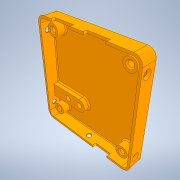
# Autodesk Inventor part: Дно корпуса электроники
Saved by Autodesk Inventor 2021.1 (Build 251245010, 245A)
## iProperties
Created: 2026-06-02
Part Number: Дно корпуса электроники
Material: Типовые
Document SubType Name: Modeling
Designer: Андрей Тарасов
Density: 1 g/cm^3
Appearance: По умолчанию
Author: Андрей Тарасов
Autodesk Inventor part; units mm, degrees
ref_plane "YZ Plane" through (0, 0, 0) normal (1, 0, 0) x (0, 1, 0)
ref_plane "XZ Plane" through (0, 0, 0) normal (0, 1, 0) x (-1, 0, 0)
ref_plane "XY Plane" through (0, 0, 0) normal (0, 0, 1) x (1, 0, 0)
sketch "Эскиз1" plane through (0, 0, 0) normal (0, 0, 1) x (1, 0, 0)
  line L0 (5, 0) -> (63.2, 0)
  line L1 (68.2, 5) -> (68.2, 65.2)
  line L2 (63.2, 70.2) -> (5, 70.2)
  line L3 (0, 65.2) -> (0, 5)
  arc A0 (5, 70.2) -> (0, 65.2) centre (5, 65.2) ccw
  arc A1 (68.2, 65.2) -> (63.2, 70.2) centre (63.2, 65.2) ccw
  arc A2 (0, 5) -> (5, 0) centre (5, 5) ccw
  arc A3 (63.2, 0) -> (68.2, 5) centre (63.2, 5) ccw
  line L4 (0, 64.1) -> (68.2, 64.1) construction
  line L5 (0, 6.1) -> (68.2, 6.1) construction
  line L6 (6.1, 70.2) -> (6.1, 0) construction
  line L7 (62.1, 70.2) -> (62.1, 0) construction
  circle A4 centre (25, 19.2) radius 1.9
  circle A5 centre (15, 19.2) radius 1.9
  line L8 (68.2, 19.2) -> (0, 19.2) construction
  point P0 (0, 0)
  point P1 (68.2, 70.2)
  point P2 (68.2, 0)
  point P3 (0, 70.2)
  dimension "d0" = 70.2
  dimension "d1" = 68.2
  dimension "d14" = 5
  dimension "d21" = 58
  dimension "d22" = 56
  dimension "d23" = 6.1
  dimension "d24" = 6.1
  dimension "d52" = 3.8
  dimension "d57" = 19.2
  dimension "d59" = 10
  dimension "d60" = 15
  constraints: 20 point on line, 18 end point, 8 point on circle, 8 tangent, 6 centre point, 6 perpendicular, 4 equal radius, 2 parallel, 1 horizontal
  measures "d0" distance of point (0, 70.2) point (0, 0)
  measures "d1" distance of point (0, 0) point (68.2, 0)
  measures "d14" radius of A0
  measures "d21" distance between parallel lines of L4 L5
  measures "d22" distance between parallel lines of L7 L6
  measures "d23" distance between parallel lines of L6 L3
  measures "d24" distance between parallel lines of L0 L5
  measures "d52" diameter of A4
  measures "d57" distance between parallel lines of L0 L8
  measures "d59" distance of A4.centre A5.centre
  measures "d60" distance from line of L3 A5.centre
extrude "Выдавливание1" add sketch "Эскиз1" along normal blind 1
sketch "Эскиз3" plane through (0, 0, 1) normal (0, 0, 1) x (1, 0, 0)
  line L0 (0, 65.2) -> (0, 5) projected
  arc A0 (0, 5) -> (5, 0) centre (5, 5) ccw projected
  line L1 (5, 0) -> (63.2, 0) projected
  arc A1 (63.2, 0) -> (68.2, 5) centre (63.2, 5) ccw projected
  line L2 (68.2, 5) -> (68.2, 65.2) projected
  arc A2 (68.2, 65.2) -> (63.2, 70.2) centre (63.2, 65.2) ccw projected
  line L3 (63.2, 70.2) -> (5, 70.2) projected
  arc A3 (5, 70.2) -> (0, 65.2) centre (5, 65.2) ccw projected
  line L4 (5, 68.6) -> (63.2, 68.6)
  arc A4 (66.6, 65.2) -> (63.2, 68.6) centre (63.2, 65.2) ccw
  line L5 (66.6, 65.2) -> (66.6, 5)
  arc A5 (63.2, 1.6) -> (66.6, 5) centre (63.2, 5) ccw
  line L6 (63.2, 1.6) -> (5, 1.6)
  arc A6 (1.6, 5) -> (5, 1.6) centre (5, 5) ccw
  line L7 (1.6, 5) -> (1.6, 65.2)
  arc A7 (5, 68.6) -> (1.6, 65.2) centre (5, 65.2) ccw
  point P0 (0, 0)
  dimension "d15" = 1.6
  constraints: 8 end point, 8 point on circle, 4 centre point, 7 other
  measures "d15" distance between parallel lines of L3 L4
extrude "Выдавливание3" add sketch "Эскиз3" along normal blind 9
chamfer "Фаска1" distance 0.6 angle 45 16 edges at (34.1, 0, 0) (66.7355, 1.4645, 0) (68.2, 35.1, 0) (66.7355, 68.7355, 0) (34.1, 70.2, 0) (1.4645, 68.7355, 0) (0, 35.1, 0) (1.4645, 1.4645, 0) (34.1, 68.6, 1) (2.5958, 67.6042, 1) (1.6, 35.1, 1) (2.5958, 2.5958, 1) (34.1, 1.6, 1) (65.6042, 2.5958, 1) (66.6, 35.1, 1) (65.6042, 67.6042, 1)
sketch "Эскиз4" plane through (5, 0, 10) normal (0, 1, 0) x (1, 0, 0)
  line L0 (0, 8.4) -> (0, 0) projected
  line L1 (58.2, 8.4) -> (58.2, 0) projected
  line L2 (0, 4.2) -> (58.2, 4.2) construction
  line L3 (58.2, 9.4) -> (58.2, 0) projected
  circle A0 centre (29.1, 4.2) radius 1.55
  point P0 (-5, 10)
  dimension "d25" = 3.1
  constraints: 2 end point, 2 midpoint, 1 centre point, 1 perpendicular, 1 point on line
  measures "d25" diameter of A0
extrude "Выдавливание4" cut sketch "Эскиз4" along normal blind 10
sketch "Эскиз5" plane through (0, 5, 10) normal (-1, 0, 0) x (0, 0, 1)
  line L0 (-8.4, 60.2) -> (0, 60.2) projected
  line L1 (-8.4, 0) -> (0, 0) projected
  line L2 (-4.2, 60.2) -> (-4.2, 0) construction
  circle A0 centre (-4.2, 55.2) radius 1.55
  circle A1 centre (-4.2, 5) radius 1.55
  point P0 (-10, -5)
  dimension "d31" = 3.1
  dimension "d41" = 5
  dimension "d42" = 5
  constraints: 2 centre point, 2 end point, 2 midpoint, 2 point on line, 1 equal radius
  measures "d31" diameter of A0
  measures "d41" distance from line of L0 A0.centre
  measures "d42" distance from line of L1 A1.centre
extrude "Выдавливание5" cut sketch "Эскиз5" against normal up to surface (68.2 mm away)
chamfer "Фаска3" distance 1.2 angle 45 5 edges at (68.2, 60.2, 4.25) (0, 60.2, 4.25) (32.55, 0, 5.8) (0, 10, 4.25) (68.2, 10, 4.25)
fillet "Сопряжение2" radius 0.2 5 edges at (1.6, 60.2, 4.25) (32.55, 1.6, 5.8) (66.6, 60.2, 4.25) (1.6, 10, 4.25) (66.6, 10, 4.25)
sketch "Эскиз6" plane through (0, 0, 10) normal (0, 0, 1) x (1, 0, 0)
  line L0 (5, 68.6) -> (63.2, 68.6) projected
  line L1 (63.2, 70.2) -> (5, 70.2) projected
  line L2 (48.2, 68.6) -> (35.2, 68.6)
  line L3 (35.2, 68.6) -> (35.2, 70.2)
  line L4 (35.2, 70.2) -> (48.2, 70.2)
  line L5 (48.2, 70.2) -> (48.2, 68.6)
  line L6 (24.8, 68.6) -> (11.8, 68.6)
  line L7 (11.8, 68.6) -> (11.8, 70.2)
  line L8 (11.8, 70.2) -> (24.8, 70.2)
  line L9 (24.8, 70.2) -> (24.8, 68.6)
  line L10 (63.2, 0) -> (5, 0) projected
  line L11 (5, 1.6) -> (63.2, 1.6) projected
  line L12 (52.2, 0) -> (42, 0)
  line L13 (42, 0) -> (42, 1.6)
  line L14 (42, 1.6) -> (52.2, 1.6)
  line L15 (52.2, 1.6) -> (52.2, 0)
  point P0 (0, 0)
  point P1 (0, 65.2)
  point P2 (68.2, 65.2)
  point P3 (11.8, 70.2)
  point P4 (0, 5)
  point P5 (68.2, 5)
  point P6 (52.2, 1.6)
  point P7 (42, 0)
  dimension "d43" = 11.8
  dimension "d44" = 20
  dimension "d45" = 13
  dimension "d46" = 13
  dimension "d49" = 42
  dimension "d50" = 16
  constraints: 24 end point, 6 parallel, 6 point on line, 3 horizontal, 3 perpendicular
  measures "d43" distance from line of point (0, 65.2) L7
  measures "d44" distance from line of point (68.2, 65.2) L5
  measures "d45" distance between parallel lines of L3 L5
  measures "d46" distance between parallel lines of L7 L9
  measures "d49" distance from line of point (0, 5) L13
  measures "d50" distance from line of point (68.2, 5) L15
extrude "Выдавливание6" cut sketch "Эскиз6" against normal blind 2.5 contours L7 L1 L9 L0 | L3 L1 L5 L0 | L10 L13 L11 L15
fillet "Сопряжение3" radius 0.8 12 edges at (52.2, 0, 8.75) (52.2, 1.6, 8.75) (42, 0, 8.75) (42, 1.6, 8.75) (11.8, 70.2, 8.75) (11.8, 68.6, 8.75) (35.2, 68.6, 8.75) (35.2, 70.2, 8.75) (48.2, 70.2, 8.75) (48.2, 68.6, 8.75) (24.8, 68.6, 8.75) (24.8, 70.2, 8.75)
sketch "Эскиз7" plane through (0, 0, 1) normal (0, 0, 1) x (1, 0, 0)
  circle A0 centre (25, 19.2) radius 4.5
  circle A1 centre (15, 19.2) radius 1.9 projected
  circle A2 centre (25, 19.2) radius 1.9 projected
  line L0 (29.5, 14.7) -> (1.6, 14.7)
  line L1 (1.6, 14.7) -> (1.6, 23.7)
  line L2 (1.6, 23.7) -> (29.5, 23.7)
  line L3 (29.5, 23.7) -> (29.5, 14.7)
  line L4 (1.6, 65.2) -> (1.6, 5) projected
  point P0 (0, 0)
  point P1 (25, 23.7)
  point P2 (25, 14.7)
  dimension "d62" = 9
  constraints: 8 end point, 3 tangent, 2 parallel, 1 centre point, 1 coincident, 1 collinear, 1 horizontal, 1 perpendicular
  measures "d62" diameter of A0
extrude "Выдавливание7" add sketch "Эскиз7" along normal blind 4 contours A0 | A0 L0 L1 L2
chamfer "Фаска4" distance 1 angle 45 5 edges at (13.1, 19.2, 0) (23.1, 19.2, 0) (13.6, 14.7, 1) (29.5, 19.2, 1) (13.6, 23.7, 1)
sketch "Эскиз8" plane through (0, 0, 1) normal (0, 0, 1) x (1, 0, 0)
  line L0 (66, 65.2) -> (66, 5) projected
  line L1 (66, 62.2) -> (2.2, 62.2) construction
  line L2 (2.2, 24.7) -> (2.2, 65.2) projected
  line L3 (66.0313, 8.2) -> (2.2, 8.2) construction
  line L4 (2.2, 5) -> (2.2, 13.7) projected
  line L5 (5, 68) -> (63.2, 68) projected
  line L6 (60, 68) -> (60, 2.2) construction
  line L7 (8, 68) -> (8, 2.2) construction
  line L8 (63.2, 2.2) -> (5, 2.2) projected
  line L9 (5, 70.2) -> (63.2, 70.2) projected
  line L10 (0, 5) -> (0, 65.2) projected
  circle A0 centre (60, 62.2) radius 1.65
  circle A1 centre (60, 8.2) radius 1.65
  circle A2 centre (8, 62.2) radius 1.65
  circle A3 centre (8, 8.2) radius 1.65
  circle A4 centre (60, 62.2) radius 4
  circle A5 centre (60, 8.2) radius 4
  circle A6 centre (8, 8.2) radius 4
  circle A7 centre (8, 62.2) radius 4
  point P0 (0, 0)
  dimension "d68" = 54
  dimension "d69" = 8
  dimension "d70" = 8
  dimension "d71" = 52
  dimension "d72" = 3.3
  dimension "d73" = 8
  constraints: 15 point on line, 8 centre point, 8 end point, 6 equal radius, 4 coincident, 2 horizontal, 2 vertical
  measures "d68" distance between parallel lines of L3 L1
  measures "d69" distance between parallel lines of L1 L9
  measures "d70" distance between parallel lines of L10 L7
  measures "d71" distance between parallel lines of L7 L6
  measures "d72" diameter of A0
  measures "d73" diameter of A4
extrude "Выдавливание8" add sketch "Эскиз8" along normal blind 6
chamfer "Фаска5" distance 0.8 angle 45 8 edges at (58.35, 62.2, 7) (58.35, 8.2, 7) (6.35, 8.2, 7) (6.35, 62.2, 7) (4, 62.2, 1) (4, 8.2, 1) (56, 8.2, 1) (56, 62.2, 1)
equation "\"d0\" = d21 + 2 * d23"
equation "\"d1\" = d22 + 2 * d24"
equation "\"d42\" = d41"
